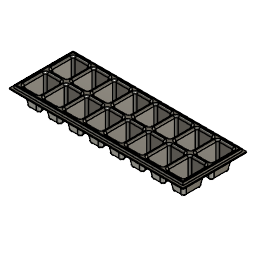
Ice Cube (Autodesk Fusion 360 design; units mm, degrees)
part number: 2026-04-19-20-25-36-678
Autodesk Fusion 360 part; units mm, degrees
sketch "Sketch1" plane through (0, 0, 0) normal (0, 0, 1) x (1, 0, 0)
  line L0 (149.315, 50.8) -> (-149.315, 50.8)
  line L1 (-149.315, 50.8) -> (-149.315, -50.8)
  line L2 (-149.315, -50.8) -> (149.315, -50.8)
  line L3 (149.315, -50.8) -> (149.315, 50.8)
  line L4 (149.315, 50.8) -> (-149.315, -50.8) construction
  line L5 (-149.315, 50.8) -> (149.315, -50.8) construction
  dimension "d1" = 101.6
  constraint horizontal L0
  constraint perpendicular L0 L1
  constraint parallel L0 L2
  constraint parallel L1 L3
  constraint coincident L4 origin
  constraint coincident L5 origin
  measures "d1" distance of L0.end L1.end
extrude "Extrude1" add sketch "Sketch1" along normal blind 50.8
sketch "Sketch2" plane through (0, 0, 50.8) normal (0, 0, 1) x (-1, 0, 0)
  line L0 (-149.315, 50.8) -> (-149.315, -50.8)
  line L1 (-149.315, -50.8) -> (149.315, -50.8)
  line L2 (149.315, -50.8) -> (149.315, 50.8)
  line L3 (149.315, 50.8) -> (-149.315, 50.8)
  line L4 (144.235, 45.72) -> (113.755, 45.72)
  line L5 (113.755, 45.72) -> (113.755, 3.81)
  line L6 (113.755, 3.81) -> (144.235, 3.81)
  line L7 (144.235, 3.81) -> (144.235, 45.72)
  line L8 (144.235, 45.72) -> (113.755, 3.81) construction
  line L9 (113.755, 45.72) -> (144.235, 3.81) construction
  point P0 (128.995, 24.765)
  dimension "d4" = 30.48
  dimension "d5" = 41.91
  dimension "d6" = 5.08
  dimension "d7" = 5.08
  constraint horizontal L4
  constraint perpendicular L4 L5
  constraint parallel L4 L6
  constraint parallel L5 L7
  constraint coincident L8 P0
  constraint coincident L9 P0
  measures "d4" distance of L5.end L6.end
  measures "d5" distance of L4.end L5.end
  measures "d6" distance of L3 L4
  measures "d7" distance of L2 L7
extrude "Extrude2" cut sketch "Sketch2" against normal blind 33.02 draft -10 contours L4 L5 L6 L7
fillet "Fillet1" radius 3.302 12 edges at (-119.5773, -24.765, 17.78) (-128.995, -9.6323, 17.78) (-138.4126, -24.765, 17.78) (-128.995, -39.8977, 17.78) (-116.6661, -42.8088, 34.29) (-141.3238, -42.8088, 34.29) (-141.3238, -6.7212, 34.29) (-116.6661, -6.7212, 34.29) (-128.995, -3.81, 50.8) (-113.755, -24.765, 50.8) (-128.995, -45.72, 50.8) (-144.235, -24.765, 50.8)
pattern_linear "R-Pattern1" count 8 spacing 37.0114 along (1, 0, 0) count 2 spacing 49.784 along (0, 1, 0) of "Extrude2", "Fillet1"
shell "Shell1" thickness 1.778 removed faces 5 at (49.7717, -50.8, 33.8667) at (-149.315, 16.9333, 33.8667) at (-49.7717, 50.8, 33.8667) at (149.315, -16.9333, 33.8667) at (-49.7717, 16.9333, 0)
sketch "Sketch3" plane through (0, 0, 0) normal (0, 1, 0) x (1, 0, 0)
  line L0 (-149.3012, -50.7626) -> (-149.3012, -44.4126)
  line L1 (-149.3012, -44.4126) -> (-155.6512, -44.4126)
  line L2 (-155.6512, -44.4126) -> (-155.6512, -46.1906)
  line L3 (-155.6512, -46.1906) -> (-151.5, -46.1906)
  line L4 (-151.5, -46.1906) -> (-151.5, -50.7335)
  line L5 (-151.5, -50.7335) -> (-149.3012, -50.7626)
  dimension "d17" = 6.35
  dimension "d18" = 6.35
  dimension "d19" = 1.778
  constraint vertical L0
  constraint perpendicular L0 L1
  constraint perpendicular L1 L2
  constraint perpendicular L2 L3
  constraint perpendicular L3 L4
  measures "d17" distance of L0.start L0.end
  measures "d18" distance of L0.end L1.end
  measures "d19" distance of L1.end L2.end
sweep "Sweep1" add profiles "Sketch3" along 4 edges at (0, 50.8, 50.8) (-149.315, 0, 50.8) (0, -50.8, 50.8) (149.315, 0, 50.8) section 1
